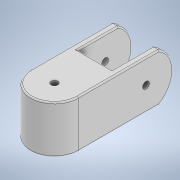
# Autodesk Inventor part: Wirst1
Saved by Autodesk Inventor 2021 (Build 250183000, 183)
## iProperties
Created: 2024-09-30
Part Number: Wirst1
Material: Generic
Document SubType Name: Modeling
Designer: Swoby
Density: 1 g/cm^3
Appearance: Default
Author: Swoby
Autodesk Inventor part; units mm, degrees
ref_plane "YZ Plane" through (0, 0, 0) normal (1, 0, 0) x (0, 1, 0)
ref_plane "XZ Plane" through (0, 0, 0) normal (0, 1, 0) x (-1, 0, 0)
ref_plane "XY Plane" through (0, 0, 0) normal (0, 0, 1) x (1, 0, 0)
sketch "Sketch1" plane through (0, 0, 0) normal (0, 1, 0) x (-1, 0, 0)
  arc A0 (35, 0) -> (-35, 0) centre (0, 0) ccw
  line L0 (35, 0) -> (-35, 0) construction
  line L1 (-35, 0) -> (-35, -139.5)
  line L2 (-35, -139.5) -> (35, -139.5)
  line L3 (35, -139.5) -> (35, 0)
  arc A1 (-35, 0) -> (35, 0) centre (0, 0) ccw construction
  line L4 (-25, -139.5) -> (25, -139.5)
  line L5 (25, -139.5) -> (25, -59.5)
  line L6 (25, -59.5) -> (-25, -59.5)
  line L7 (-25, -59.5) -> (-25, -139.5)
  circle A2 centre (0, 0) radius 5
  point P0 (25, -139.5)
  dimension "d0" = 70
  dimension "d1" = 139.5
  dimension "d2" = 10
  dimension "d3" = 10
  dimension "d4" = 80
  dimension "d11" = 10
  constraints: 16 end point, 4 parallel, 4 point on circle, 3 centre point, 2 coincident, 2 horizontal, 2 perpendicular, 2 tangent, 1 point on line
  measures "d0" diameter of A0
  measures "d1" distance of L2.end L0.start
  measures "d2" distance between parallel lines of L5 L3
  measures "d3" distance between parallel lines of L1 L7
  measures "d4" distance between parallel lines of L2 L6
  measures "d11" diameter of A2
extrude "Extrusion1" add sketch "Sketch1" along normal blind 70 contours L3 L2 L5 L6 L7 L1 A0
sketch "Sketch2" plane through (35, 0, 0) normal (1, 0, 0) x (0, 0, -1)
  line L0 (0, 0) -> (139.5, 0) projected
  line L1 (139.5, 0) -> (139.5, 70) projected
  line L2 (0, 70) -> (139.5, 70) projected
  line L3 (0, 0) -> (0, 70) projected
  arc A0 (118.8649, 70) -> (118.8649, 0) centre (99.5, 35) ccw
  line L4 (99.5, 35) -> (139.5, 35)
  arc A1 (139.5, 35) -> (118.8649, 70) centre (99.5, 35) ccw
  arc A2 (118.8649, 0) -> (139.5, 35) centre (99.5, 35) ccw
  circle A3 centre (99.5, 35) radius 5
  point P0 (0, 0)
  dimension "d7" = 80
  dimension "d8" = 10
  constraints: 6 point on circle, 4 centre point, 2 end point, 2 point on line, 1 coincident, 1 horizontal, 1 midpoint
  measures "d7" diameter of A0
  measures "d8" diameter of A3
extrude "Extrusion2" cut sketch "Sketch2" against normal through all contours A2 L1 L0 | A3 | A1 L2 L1
fillet "Fillet1" radius 2 16 edges at (0, 70, 35) (-35, 70, -59.4325) (35, 70, -59.4325) (0, 0, 35) (-35, 0, -59.4325) (35, 0, -59.4325) (-25, 35, -139.5) (35, 35, -139.5) (25, 35, -139.5) (-35, 35, -139.5) (-25, 70, -89.1825) (0, 70, -59.5) (0, 0, -59.5) (25, 0, -89.1825) (25, 70, -89.1825) (-25, 0, -89.1825)
body "Solid1"
